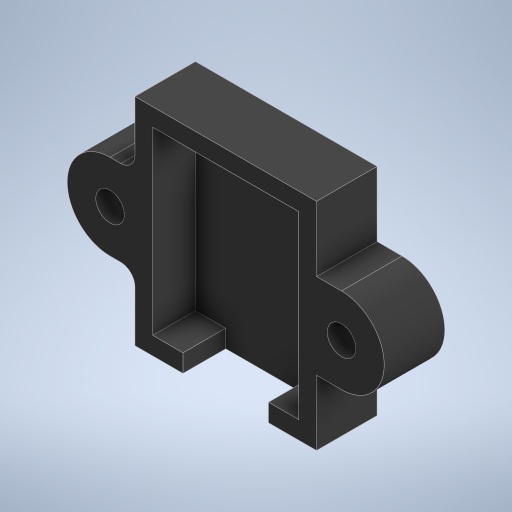
# Autodesk Inventor part: KeyPad_Holder
Saved by Autodesk Inventor 2023 (Build 270158000, 158)
## iProperties
Created: 2024-08-01
Part Number: KeyPad_Holder
Material: Generic
Document SubType Name: Modeling
Designer: Swoby
Density: 1 g/cm^3
Appearance: Default
Author: Swoby
Autodesk Inventor part; units mm, degrees
ref_plane "YZ Plane" through (0, 0, 0) normal (1, 0, 0) x (0, 1, 0)
ref_plane "XZ Plane" through (0, 0, 0) normal (0, 1, 0) x (-1, 0, 0)
ref_plane "XY Plane" through (0, 0, 0) normal (0, 0, 1) x (1, 0, 0)
sketch "Sketch1" plane through (0, 0, 0) normal (0, 0, 1) x (1, 0, 0)
  line L0 (-10.25, -12.65) -> (10.25, -12.65)
  line L1 (10.25, -12.65) -> (10.25, 12.65)
  line L2 (10.25, 12.65) -> (-10.25, 12.65)
  line L3 (-10.25, 12.65) -> (-10.25, -12.65)
  line L4 (-10.25, -12.65) -> (10.25, 12.65) construction
  line L5 (10.25, -12.65) -> (-10.25, 12.65) construction
  line L6 (-12.75, -15.15) -> (12.75, -15.15)
  line L7 (12.75, -15.15) -> (12.75, 15.15)
  line L8 (12.75, 15.15) -> (-12.75, 15.15)
  line L9 (-12.75, 15.15) -> (-12.75, -15.15)
  line L10 (-6, -15.15) -> (6, -15.15)
  line L11 (6, -15.15) -> (6, -12.65)
  line L12 (6, -12.65) -> (-6, -12.65)
  line L13 (-6, -12.65) -> (-6, -15.15)
  line L14 (-10.25, 0) -> (10.25, 0) construction
  circle A0 centre (-16.25, 0) radius 2
  arc A1 (-16.25, 6) -> (-16.25, -6) centre (-16.25, 0) ccw
  line L15 (-16.25, 6) -> (-12.75, 6)
  line L16 (-16.25, -6) -> (-12.75, -6)
  circle A2 centre (16.25, 0) radius 2
  line L17 (16.25, 6) -> (12.75, 6)
  line L18 (16.25, -6) -> (12.75, -6)
  arc A3 (16.25, -6) -> (16.25, 6) centre (16.25, 0) ccw
  point P0 (0, 0)
  point P1 (0, -12.65)
  dimension "d0" = 20.5
  dimension "d1" = 25.3
  dimension "d2" = 2.5
  dimension "d3" = 12
  dimension "d18" = 4
  dimension "d20" = 3.5
  dimension "d21" = 12
  dimension "d24" = 4
  dimension "d26" = 3.5
  dimension "d27" = 6
  constraints: 38 end point, 8 point on line, 6 midpoint, 6 parallel, 5 perpendicular, 4 centre point, 4 horizontal, 4 point on circle, 4 tangent, 2 coincident, 3 other
  measures "d0" distance of L1.end L2.end
  measures "d1" distance of L0.end L1.end
  measures "d2" distance between parallel lines of L3 L9
  measures "d3" distance between parallel lines of L11 L13
  measures "d18" diameter of A0
  measures "d20" distance from line of L9 A0.centre
  measures "d21" diameter of A1
  measures "d24" diameter of A2
  measures "d26" distance from line of L7 A2.centre
  measures "d27" radius of A3
extrude "Extrusion1" add sketch "Sketch1" against normal blind 2.5
extrude "Extrusion2" add sketch "Sketch1" along normal blind 6 contours L0 L13 L6 L9 L8 L7 L11 L1 L2 L3 | L16 A1 L15 L9 | L7 L17 A3 L18
fillet "Fillet1" radius 2 2 edges at (-12.75, -6, 1.75) (-12.75, 6, 1.75)
sketch "Sketch2" plane through (0, 0, -2.5) normal (0, 0, -1) x (-1, 0, 0)
  circle A0 centre (16.25, 0) radius 2
  line L0 (-12.9, 1.9341) -> (-12.9, -1.9341)
  line L1 (-12.9, -1.9341) -> (-16.25, -3.8682)
  line L2 (-16.25, -3.8682) -> (-19.6, -1.9341)
  line L3 (-19.6, -1.9341) -> (-19.6, 1.9341)
  line L4 (-19.6, 1.9341) -> (-16.25, 3.8682)
  line L5 (-16.25, 3.8682) -> (-12.9, 1.9341)
  line L6 (12.9, 1.9341) -> (16.25, 3.8682)
  line L7 (16.25, 3.8682) -> (19.6, 1.9341)
  line L8 (19.6, 1.9341) -> (19.6, -1.9341)
  line L9 (19.6, -1.9341) -> (16.25, -3.8682)
  line L10 (16.25, -3.8682) -> (12.9, -1.9341)
  line L11 (12.9, -1.9341) -> (12.9, 1.9341)
  line L12 (-12.75, 15.15) -> (-12.75, -15.15) projected
  circle A1 centre (-16.25, 0) radius 2 projected
  circle A2 centre (-16.25, 0) radius 2 projected
  circle A3 centre (16.25, 0) radius 2 projected
  circle A4 centre (16.25, 0) radius 2 projected
  point P0 (0, 0)
  point P1 (-16.25, 0)
  point P2 (-12.75, 5.5)
  dimension "d13" = 6.7
  dimension "d14" = 6.7
  constraints: 24 end point, 3 coincident, 2 parallel, 1 centre point, 26 other
  measures "d13" distance between parallel lines of L1 L4
  measures "d14" distance between parallel lines of L9 L6
extrude "Extrusion3" cut sketch "Sketch2" against normal blind 3 contours A0 | L0 L1 L2 L3 L4 L5 | L6 L7 L8 L9 L10 L11 | A1
body "Solid1"
